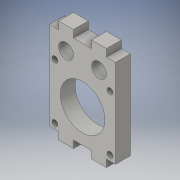
# Autodesk Inventor part: Motor Bracket
Saved by Autodesk Inventor 2016 (Build 200138000, 138)
## iProperties
Created: 2016-04-23
Part Number: Motor Bracket
Material: Generic
Document SubType Name: Modeling
Designer: rubenjm
Density: 1 g/cm^3
Appearance: Default
Author: rubenjm
Autodesk Inventor part; units mm, degrees
ref_plane "YZ Plane" through (0, 0, 0) normal (1, 0, 0) x (0, 1, 0)
ref_plane "XZ Plane" through (0, 0, 0) normal (0, 1, 0) x (-1, 0, 0)
ref_plane "XY Plane" through (0, 0, 0) normal (0, 0, 1) x (1, 0, 0)
sketch "Sketch1" plane through (0, 0, 0) normal (0, 0, 1) x (1, 0, 0)
  line L0 (56.388, 0) -> (56.388, 75.438)
  line L1 (0, 75.438) -> (0, 0)
  circle A0 centre (28.194, 28.194) radius 19.05
  line L2 (0, 75.438) -> (4.6228, 75.438) construction
  line L3 (4.6228, 75.438) -> (4.6228, 70.8152) construction
  line L4 (4.6228, 70.8152) -> (0, 70.8152) construction
  line L5 (0, 70.8152) -> (0, 75.438) construction
  line L6 (28.194, 75.438) -> (28.194, 0) construction
  line L7 (56.388, 37.719) -> (0, 37.719) construction
  line L8 (28.194, 75.438) -> (0, 75.438) construction
  line L9 (28.194, 75.438) -> (0, 75.438) construction
  line L10 (14.097, 75.438) -> (14.097, 78.613) construction
  line L11 (7.747, 81.788) -> (20.447, 81.788)
  line L12 (20.447, 81.788) -> (20.447, 75.438)
  line L13 (7.747, 75.438) -> (7.747, 81.788)
  line L14 (7.747, 81.788) -> (20.447, 75.438) construction
  line L15 (20.447, 81.788) -> (7.747, 75.438) construction
  line L16 (7.747, 75.438) -> (0, 75.438)
  line L17 (42.291, 75.438) -> (42.291, 78.613) construction
  line L18 (48.641, 81.788) -> (35.941, 81.788)
  line L19 (35.941, 81.788) -> (35.941, 75.438)
  line L20 (48.641, 75.438) -> (48.641, 81.788)
  line L21 (48.641, 81.788) -> (35.941, 75.438) construction
  line L22 (35.941, 81.788) -> (48.641, 75.438) construction
  line L23 (56.388, 75.438) -> (48.641, 75.438)
  line L24 (35.941, 75.438) -> (20.447, 75.438)
  line L25 (14.097, 0) -> (14.097, -3.175) construction
  line L26 (7.747, -6.35) -> (20.447, -6.35)
  line L27 (20.447, -6.35) -> (20.447, 0)
  line L28 (7.747, 0) -> (7.747, -6.35)
  line L29 (7.747, -6.35) -> (20.447, 0) construction
  line L30 (20.447, -6.35) -> (7.747, 0) construction
  line L31 (42.291, 0) -> (42.291, -3.175) construction
  line L32 (48.641, -6.35) -> (35.941, -6.35)
  line L33 (35.941, -6.35) -> (35.941, 0)
  line L34 (48.641, -6.35) -> (35.941, 0) construction
  line L35 (35.941, -6.35) -> (48.641, 0) construction
  line L36 (48.641, 0) -> (48.641, -6.35)
  line L37 (0, 0) -> (7.747, 0)
  line L38 (20.447, 0) -> (35.941, 0)
  line L39 (48.641, 0) -> (56.388, 0)
  line L40 (56.394, -0.006) -> (-0.006, -0.006) construction
  line L41 (-0.006, -0.006) -> (-0.006, 56.394) construction
  line L42 (-0.006, 56.394) -> (56.394, 56.394) construction
  line L43 (0, 56.4) -> (0, 0) construction
  line L44 (-0.006, -0.006) -> (56.394, 56.394) construction
  line L45 (51.764, 4.624) -> (4.624, 4.624) construction
  line L46 (4.624, 4.624) -> (4.624, 51.764) construction
  line L47 (4.624, 51.764) -> (51.764, 51.764) construction
  line L48 (51.764, 51.764) -> (51.764, 4.624) construction
  line L49 (51.764, 4.624) -> (4.624, 51.764) construction
  line L50 (4.624, 4.624) -> (51.764, 51.764) construction
  circle A1 centre (4.5934, 4.5934) radius 2.5
  circle A2 centre (4.624, 51.764) radius 2.5
  circle A3 centre (51.764, 51.764) radius 2.5
  circle A4 centre (51.764, 4.624) radius 2.5
  point P0 (28.194, 28.194)
  dimension "d0" = 75.438
  dimension "d1" = 56.388
  dimension "d2" = 38.1
  dimension "d8" = 4.6228
  dimension "d16" = 3.175
  dimension "d18" = 12.7
  dimension "d19" = 47.14
  dimension "d20" = 47.14
  dimension "d21" = 5
  dimension "d22" = 5
  dimension "d23" = 5
  dimension "d24" = 5
  constraints: 102 end point, 18 symmetric about line, 17 parallel, 16 midpoint, 9 horizontal, 7 perpendicular, 5 centre point, 3 coincident, 2 point on line, 1 vertical
  measures "d0" distance of L0.start L0.end
  measures "d1" distance of L0.end L1.start
  measures "d2" diameter of A0
  measures "d8" distance of L2.end L3.end
  measures "d16" distance of L10.start L10.end
  measures "d18" distance of L13.start L12.end
  measures "d19" distance of L46.end L47.end
  measures "d20" distance of L45.end L46.end
  measures "d21" diameter of A1
  measures "d22" diameter of A2
  measures "d23" diameter of A3
  measures "d24" diameter of A4
extrude "Extrusion2" add sketch "Sketch1" along normal blind 12.7
sketch "Sketch2" plane through (0, 0, 12.7) normal (0, 0, 1) x (1, 0, 0)
  line L0 (0, 0) -> (0, 75.438) construction
  line L1 (0, 75.438) -> (0, 62.738) construction
  line L2 (0, 75.438) -> (12.7, 75.438) construction
  line L3 (0, 62.738) -> (56.388, 62.738) construction
  line L4 (28.194, 62.738) -> (0, 62.738) construction
  circle A0 centre (14.097, 62.738) radius 6.35
  line L5 (28.194, 62.738) -> (28.194, 75.438) construction
  circle A1 centre (42.291, 62.738) radius 6.35
  dimension "d27" = 12.7
  dimension "d28" = 90
  dimension "d29" = 56.388
  dimension "d30" = 90
  dimension "d31" = 12.7
  constraints: 10 end point, 3 perpendicular, 2 centre point, 2 midpoint, 1 collinear, 1 horizontal, 1 symmetric about line, 1 vertical, 1 other
  measures "d27" distance of L0.end L1.end
  measures "d28" angle of L1 L2
  measures "d29" distance of L1.end L3.end
  measures "d30" angle of L3 L1
  measures "d31" diameter of A0
extrude "Extrusion3" cut sketch "Sketch2" against normal through all
body "Solid2"
